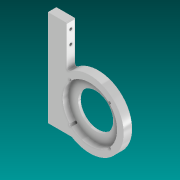
# Autodesk Inventor part: motorFrame
Saved by Autodesk Inventor 2020.3 (Build 243373000, 373)
## iProperties
Created: 2020-05-19
Part Number: motorFrame
Material: Aluminum 6061
Document SubType Name: Modeling
Designer: Svend
Density: 2.7 g/cm^3
Appearance: Aluminum - Polished
Author: Svend
Autodesk Inventor part; units mm, degrees
ref_plane "YZ Plane" through (0, 0, 0) normal (1, 0, 0) x (0, 1, 0)
ref_plane "XZ Plane" through (0, 0, 0) normal (0, 1, 0) x (-1, 0, 0)
ref_plane "Work Plane1" through (0, 0, 0) normal (0, 0, 1) x (1, 0, 0)
sketch "Sketch1" plane through (0, 0, 0) normal (0, 0, 1) x (1, 0, 0)
  circle A0 centre (0, 0) radius 21 projected
  circle A1 centre (23.57, -23.57) radius 2 projected
  circle A2 centre (23.57, 23.57) radius 2 projected
  circle A3 centre (-23.57, -23.57) radius 2.5 projected
  circle A4 centre (-23.57, 23.57) radius 2 projected
  circle A5 centre (-23.57, -23.57) radius 2 projected
  circle A6 centre (0, 0) radius 19 projected
  circle A7 centre (-23.57, 23.57) radius 2.5 projected
  circle A8 centre (-23.57, -23.57) radius 2.5 projected
  arc A9 (-29.95, -24.95) -> (-24.95, -29.95) centre (-24.95, -24.95) ccw projected
  line L0 (24.95, -29.95) -> (-24.95, -29.95) projected
  arc A10 (24.95, -29.95) -> (29.95, -24.95) centre (24.95, -24.95) ccw projected
  line L1 (29.95, 24.95) -> (29.95, -24.95) projected
  arc A11 (29.95, 24.95) -> (24.95, 29.95) centre (24.95, 24.95) ccw projected
  line L2 (-24.95, 29.95) -> (24.95, 29.95) projected
  arc A12 (-24.95, 29.95) -> (-29.95, 24.95) centre (-24.95, 24.95) ccw projected
  line L3 (-29.95, -24.95) -> (-29.95, 24.95) projected
  circle A13 centre (23.57, -23.57) radius 2.5 projected
  circle A14 centre (23.57, 23.57) radius 2.5 projected
  line L4 (-49.95, -90) -> (-49.95, 90) projected
  line L5 (-59.95, -90) -> (-49.95, -90)
  line L6 (-59.95, 90) -> (-49.95, 90)
  line L7 (40.2846, 0) -> (-40.2846, 0)
  line L8 (-49.95, -90) -> (-49.95, 90) projected
  line L9 (-59.95, -90) -> (-49.95, -90)
  line L10 (-49.95, 35.5095) -> (-26.95, 35.5095) projected
  line L11 (-24.95, 29.95) -> (-49.95, 29.95)
  line L12 (-24.95, -29.95) -> (-49.95, -29.95)
  circle A15 centre (0, 0) radius 22
  line L13 (-32.95, 22) -> (-32.95, -22) projected
  line L14 (-30.95, -14.95) -> (-49.95, -14.95)
  line L15 (-30.95, 14.95) -> (-49.95, 14.95)
  line L16 (-30.95, -14.95) -> (-30.95, 14.95)
  line L17 (24.7214, -34.026) -> (0, -42.0585)
  line L18 (0, -42.0585) -> (-24.7214, -34.026)
  line L19 (-24.7214, -34.026) -> (-40, -12.9968)
  line L20 (-40, -12.9968) -> (-40, 12.9968)
  line L21 (-40, 12.9968) -> (-24.7214, 34.026)
  line L22 (-24.7214, 34.026) -> (0, 42.0585)
  line L23 (0, 42.0585) -> (24.7214, 34.026)
  line L24 (24.7214, 34.026) -> (40, 12.9968)
  line L25 (40, 12.9968) -> (40, -12.9968)
  line L26 (40, -12.9968) -> (24.7214, -34.026)
  line L27 (-24.7214, -34.026) -> (-49.95, -34.026)
  line L28 (-24.7214, 34.026) -> (-49.95, 34.026)
  arc A16 (-24.7214, -34.026) -> (-24.7214, 34.026) centre (0, 0) ccw projected
  line L29 (-24.7214, 34.026) -> (-27.8, 34.026) projected
  line L30 (-27.8, 34.026) -> (-27.8, 80.5095) projected
  line L31 (-27.8, 80.5095) -> (-49.95, 80.5095) projected
  line L32 (-49.95, 80.5095) -> (-49.95, 14.95) projected
  line L33 (-49.95, 14.95) -> (-35.95, 14.95) projected
  arc A17 (-30.95, 9.95) -> (-35.95, 14.95) centre (-35.95, 9.95) ccw projected
  line L34 (-30.95, 9.95) -> (-30.95, -9.95) projected
  arc A18 (-35.95, -14.95) -> (-30.95, -9.95) centre (-35.95, -9.95) ccw projected
  line L35 (-35.95, -14.95) -> (-49.95, -14.95) projected
  line L36 (-49.95, -14.95) -> (-49.95, -34.026) projected
  line L37 (-49.95, -34.026) -> (-24.7214, -34.026) projected
  circle A19 centre (15.9909, -0.539) radius 1.6 projected
  circle A20 centre (-11.6884, -10.9261) radius 2 projected
  circle A21 centre (11.6884, 10.9261) radius 2 projected
  circle A22 centre (10.9261, -11.6884) radius 2 projected
  circle A23 centre (-15.9909, 0.539) radius 1.6 projected
  circle A24 centre (-0.539, -15.9909) radius 1.6 projected
  circle A25 centre (0, 0) radius 12.5 projected
  circle A26 centre (0.539, 15.9909) radius 1.6 projected
  circle A27 centre (-10.9261, 11.6884) radius 2 projected
  point P0 (0, 0)
  point P1 (-23.2856, -45.1645)
  point P2 (-49.95, -75.9684)
  point P3 (-23.2856, 45.1645)
  point P4 (-49.95, -14.95)
  point P5 (-32.95, 13.95)
  point P6 (-32.95, 14.95)
  dimension "d9" = 1
  dimension "d10" = 15
  dimension "d11" = 15
  dimension "d12" = 1
  dimension "d13" = 40
  constraints: 42 end point, 7 horizontal, 5 parallel, 2 perpendicular, 1 centre point, 1 coincident, 1 midpoint, 1 point on line, 1 symmetric about line, 1 vertical, 30 other
  measures "d9" radial gap between concentric circles of A0 A15
  measures "d10" distance between parallel lines of L12 L14
  measures "d11" distance between parallel lines of L11 L15
  measures "d12" distance between parallel lines of L3 L16
  measures "d13" distance from line of L25 point (0, 0)
extrude "Extrusion1" add sketch "Sketch1" along normal blind 10 contours L7 A15 A0 | A0 L7 A15 | A15 L7 L3 A12 L2 A11 L1 | L7 L1 A10 L0 A9 L3 A15 | L7 L25 L26 L17 L18 L19 L12 L0 A10 L1 | L1 A11 L2 L11 L21 L22 L23 L24 L25 L7 | L7 L16 L15 L21 L11 A12 L3 | L3 A9 L12 L19 L14 L16 L7 | L25 A16 | L16 A18 L13 L7 | L7 L13 A17 L16 | L24 A16 | A16 L26 | L13 A18 L14 L19 L20 L7 | L7 L20 L21 L15 A17 L13 | L16 L14 L13 A18 | A17 L13 L15 L16 | L23 A16 | A16 L17 | L19 L27 L4 L12 | L12 L4 L14 L19 | L21 L15 L4 L11 | L11 L4 L28 L21 | L20 L19 L14 L4 L15 L21 | A17 L15 L13 | L13 L14 A18 | L22 A16 | A16 L18 | A1 | A2 | A3 | A4 | A5 | A7 | A13 | A14
sketch "Sketch2" plane through (-49.95, -34.026, 0) normal (-1, 0, 0) x (0, 0, 1)
  line L0 (0, 68.0521) -> (0, 0) projected
  line L1 (0, 0) -> (10, 0) projected
  line L2 (10, 68.0521) -> (10, 0) projected
  line L3 (0, 68.0521) -> (0, 0) projected
  line L4 (10, 68.0521) -> (10, 0) projected
  line L5 (0, 68.0521) -> (10, 68.0521) projected
  line L6 (0, 0) -> (10, 0) projected
  line L7 (0, 68.0521) -> (10, 68.0521) projected
  point P0 (0, 34.026)
  point P1 (5, 7.5)
  point P2 (5, 60.5521)
  point P3 (5, 68.0521)
  point P4 (5, 19.076)
  dimension "d24" = 7.5
  dimension "d25" = 7.5
  constraints: 2 vertical alignment, 1 midpoint
  measures "d24" distance from line of L1 point (5, 7.5)
  measures "d25" distance from line of L5 point (5, 60.552)
hole "Hole1" at (-49.95, 26.526, 5) at (-49.95, -26.526, 5) direction (1, 0, 0) diameter 3.242 depth 15 tip angle 118 thread size "M4x0.7" class "6H" standard "ISO Metric profile"
sketch "Sketch3" plane through (0, 0, 10) normal (0, 0, 1) x (1, 0, 0)
  arc A0 (-24.7214, -34.026) -> (-24.7214, 34.026) centre (0, 0) ccw projected
  line L0 (-24.7214, 34.026) -> (-27.8, 34.026) projected
  line L1 (-27.8, 34.026) -> (-27.8, 80.5095) projected
  line L2 (-27.8, 80.5095) -> (-49.95, 80.5095) projected
  line L3 (-49.95, 80.5095) -> (-49.95, 14.95) projected
  line L4 (-49.95, 14.95) -> (-35.95, 14.95) projected
  arc A1 (-30.95, 9.95) -> (-35.95, 14.95) centre (-35.95, 9.95) ccw projected
  line L5 (-30.95, 9.95) -> (-30.95, -9.95) projected
  arc A2 (-35.95, -14.95) -> (-30.95, -9.95) centre (-35.95, -9.95) ccw projected
  line L6 (-35.95, -14.95) -> (-49.95, -14.95) projected
  line L7 (-49.95, -14.95) -> (-49.95, -34.026) projected
  line L8 (-49.95, -34.026) -> (-24.7214, -34.026) projected
  circle A3 centre (15.9909, -0.539) radius 1.6 projected
  circle A4 centre (-11.6884, -10.9261) radius 2 projected
  circle A5 centre (11.6884, 10.9261) radius 2 projected
  circle A6 centre (10.9261, -11.6884) radius 2 projected
  circle A7 centre (-15.9909, 0.539) radius 1.6 projected
  circle A8 centre (-0.539, -15.9909) radius 1.6 projected
  circle A9 centre (0, 0) radius 12.5 projected
  circle A10 centre (0.539, 15.9909) radius 1.6 projected
  circle A11 centre (-10.9261, 11.6884) radius 2 projected
  circle A12 centre (0, 0) radius 19 projected
  circle A13 centre (-23.57, 23.57) radius 2.5 projected
  circle A14 centre (-23.57, -23.57) radius 2.5 projected
  arc A15 (-29.95, -24.95) -> (-24.95, -29.95) centre (-24.95, -24.95) ccw projected
  line L9 (24.95, -29.95) -> (-24.95, -29.95) projected
  arc A16 (24.95, -29.95) -> (29.95, -24.95) centre (24.95, -24.95) ccw projected
  line L10 (29.95, 24.95) -> (29.95, -24.95) projected
  arc A17 (29.95, 24.95) -> (24.95, 29.95) centre (24.95, 24.95) ccw projected
  line L11 (-24.95, 29.95) -> (24.95, 29.95) projected
  arc A18 (-24.95, 29.95) -> (-29.95, 24.95) centre (-24.95, 24.95) ccw projected
  line L12 (-29.95, -24.95) -> (-29.95, 24.95) projected
  circle A19 centre (23.57, -23.57) radius 2.5 projected
  circle A20 centre (23.57, 23.57) radius 2.5 projected
  arc A21 (-37.4079, -14.95) -> (-37.4079, 14.95) centre (0, 0) ccw
  line L13 (-27.8, 34.026) -> (-27.8, 29.155)
  line L14 (-49.95, -34.026) -> (-21.5657, -34.026)
  line L15 (-49.95, -34.026) -> (-24.7214, -34.026) projected
  point P0 (0, 0)
  point P1 (-24.7214, -34.026)
  constraints: 4 end point, 4 point on circle, 2 collinear, 2 point on line, 1 centre point, 1 coincident, 1 tangent
extrude "Extrusion2" cut sketch "Sketch3" against normal blind 10 contours L14 A21 L13 L0 A0
sketch "Sketch4" plane through (0, 0, 10) normal (0, 0, 1) x (1, 0, 0)
  arc A0 (-24.7214, -34.026) -> (-24.7214, 34.026) centre (0, 0) ccw projected
  line L0 (-24.7214, 34.026) -> (-27.8, 34.026) projected
  line L1 (-27.8, 34.026) -> (-27.8, 80.5095) projected
  line L2 (-27.8, 80.5095) -> (-49.95, 80.5095) projected
  line L3 (-49.95, 80.5095) -> (-49.95, 14.95) projected
  line L4 (-49.95, 14.95) -> (-35.95, 14.95) projected
  arc A1 (-30.95, 9.95) -> (-35.95, 14.95) centre (-35.95, 9.95) ccw projected
  line L5 (-30.95, 9.95) -> (-30.95, -9.95) projected
  arc A2 (-35.95, -14.95) -> (-30.95, -9.95) centre (-35.95, -9.95) ccw projected
  line L6 (-35.95, -14.95) -> (-49.95, -14.95) projected
  line L7 (-49.95, -14.95) -> (-49.95, -34.026) projected
  line L8 (-49.95, -34.026) -> (-24.7214, -34.026) projected
  circle A3 centre (15.9909, -0.539) radius 1.6 projected
  circle A4 centre (-11.6884, -10.9261) radius 2 projected
  circle A5 centre (11.6884, 10.9261) radius 2 projected
  circle A6 centre (10.9261, -11.6884) radius 2 projected
  circle A7 centre (-15.9909, 0.539) radius 1.6 projected
  circle A8 centre (-0.539, -15.9909) radius 1.6 projected
  circle A9 centre (0, 0) radius 12.5 projected
  circle A10 centre (0.539, 15.9909) radius 1.6 projected
  circle A11 centre (-10.9261, 11.6884) radius 2 projected
  line L9 (-49.95, -90) -> (-49.95, 90) projected
  line L10 (-59.95, 90) -> (-49.95, 90)
  line L11 (-49.95, -90) -> (-49.95, 90) projected
  line L12 (-27.8, 29.155) -> (-27.8, 34.026) projected
  line L13 (-27.8, 34.026) -> (-49.95, 34.026) projected
  line L14 (-49.95, 34.026) -> (-49.95, -34.026) projected
  line L15 (-49.95, -34.026) -> (-21.5657, -34.026) projected
  arc A12 (-21.5657, -34.026) -> (-27.8, 29.155) centre (0, 0) ccw projected
  circle A13 centre (0, 0) radius 21 projected
  point P0 (0, 0)
  constraints: 2 end point, 1 horizontal, 1 other
extrude "Extrusion3" add sketch "Sketch4" against normal blind 10 contours L13 L3 L2 L1
fillet "Fillet1" radius 2 2 edges at (-27.8, 29.155, 5) (-21.5657, -34.026, 5)
fillet "Fillet2" radius 1 1 edges at (-27.8, 80.5095, 5)
sketch "Sketch5" plane through (-27.8, 33.5015, 10) normal (1, 0, 0) x (0, 0, -1)
  arc A0 (8, 9.19) -> (10, 11.19) centre (8, 11.19) ccw projected
  line L0 (10, 49.19) -> (10, 11.19) projected
  arc A1 (10, 49.19) -> (8, 51.19) centre (8, 49.19) ccw projected
  line L1 (-60.5, 51.19) -> (8, 51.19) projected
  arc A2 (-60.5, 51.19) -> (-62.5, 49.19) centre (-60.5, 49.19) ccw projected
  line L2 (-62.5, 11.19) -> (-62.5, 49.19) projected
  arc A3 (-62.5, 11.19) -> (-60.5, 9.19) centre (-60.5, 11.19) ccw projected
  line L3 (8, 9.19) -> (-60.5, 9.19) projected
  circle A4 centre (-26.25, 30.19) radius 12.6 projected
  circle A5 centre (-26.25, 14.19) radius 2 projected
  arc A6 (-59.6, 14.79) -> (-55.4, 14.79) centre (-57.5, 14.79) ccw projected
  line L4 (-59.6, 45.59) -> (-59.6, 14.79) projected
  arc A7 (-55.4, 45.59) -> (-59.6, 45.59) centre (-57.5, 45.59) ccw projected
  line L5 (-55.4, 14.79) -> (-55.4, 45.59) projected
  circle A8 centre (-42.25, 30.19) radius 2 projected
  circle A9 centre (-37.5637, 18.8763) radius 1.5 projected
  circle A10 centre (-37.5637, 41.5037) radius 1.5 projected
  circle A11 centre (-14.9363, 18.8763) radius 1.5 projected
  arc A12 (7.1, 45.59) -> (2.9, 45.59) centre (5, 45.59) ccw projected
  line L6 (7.1, 14.79) -> (7.1, 45.59) projected
  arc A13 (2.9, 14.79) -> (7.1, 14.79) centre (5, 14.79) ccw projected
  line L7 (2.9, 45.59) -> (2.9, 14.79) projected
  circle A14 centre (-10.25, 30.19) radius 2 projected
  circle A15 centre (-14.9363, 41.5037) radius 1.5 projected
  circle A16 centre (-26.25, 46.19) radius 2 projected
  circle A17 centre (-57.5, 11.46) radius 1.621 projected
  circle A18 centre (-57.5, 26.86) radius 1.621 projected
  arc A19 (8, 9.19) -> (10, 11.19) centre (8, 11.19) ccw projected
  line L8 (10, 49.19) -> (10, 11.19) projected
  arc A20 (10, 49.19) -> (8, 51.19) centre (8, 49.19) ccw projected
  line L9 (-60.5, 51.19) -> (8, 51.19) projected
  arc A21 (-60.5, 51.19) -> (-62.5, 49.19) centre (-60.5, 49.19) ccw projected
  line L10 (-62.5, 11.19) -> (-62.5, 49.19) projected
  arc A22 (-62.5, 11.19) -> (-60.5, 9.19) centre (-60.5, 11.19) ccw projected
  line L11 (8, 9.19) -> (-60.5, 9.19) projected
  circle A23 centre (-26.25, 30.19) radius 12.6 projected
  circle A24 centre (-26.25, 14.19) radius 2 projected
  arc A25 (-59.6, 14.79) -> (-55.4, 14.79) centre (-57.5, 14.79) ccw projected
  line L12 (-59.6, 45.59) -> (-59.6, 14.79) projected
  arc A26 (-55.4, 45.59) -> (-59.6, 45.59) centre (-57.5, 45.59) ccw projected
  line L13 (-55.4, 14.79) -> (-55.4, 45.59) projected
  circle A27 centre (-42.25, 30.19) radius 2 projected
  circle A28 centre (-37.5637, 18.8763) radius 1.5 projected
  circle A29 centre (-37.5637, 41.5037) radius 1.5 projected
  circle A30 centre (-14.9363, 18.8763) radius 1.5 projected
  arc A31 (7.1, 45.59) -> (2.9, 45.59) centre (5, 45.59) ccw projected
  line L14 (7.1, 14.79) -> (7.1, 45.59) projected
  arc A32 (2.9, 14.79) -> (7.1, 14.79) centre (5, 14.79) ccw projected
  line L15 (2.9, 45.59) -> (2.9, 14.79) projected
  circle A33 centre (-10.25, 30.19) radius 2 projected
  circle A34 centre (-14.9363, 41.5037) radius 1.5 projected
  circle A35 centre (-26.25, 46.19) radius 2 projected
  arc A36 (8, 9.19) -> (10, 11.19) centre (8, 11.19) ccw projected
  line L16 (10, 49.19) -> (10, 11.19) projected
  arc A37 (10, 49.19) -> (8, 51.19) centre (8, 49.19) ccw projected
  line L17 (-60.5, 51.19) -> (8, 51.19) projected
  arc A38 (-60.5, 51.19) -> (-62.5, 49.19) centre (-60.5, 49.19) ccw projected
  line L18 (-62.5, 11.19) -> (-62.5, 49.19) projected
  arc A39 (-62.5, 11.19) -> (-60.5, 9.19) centre (-60.5, 11.19) ccw projected
  line L19 (8, 9.19) -> (-60.5, 9.19) projected
  circle A40 centre (-26.25, 30.19) radius 12.6 projected
  circle A41 centre (-26.25, 14.19) radius 2 projected
  arc A42 (-59.6, 14.79) -> (-55.4, 14.79) centre (-57.5, 14.79) ccw projected
  line L20 (-59.6, 45.59) -> (-59.6, 14.79) projected
  arc A43 (-55.4, 45.59) -> (-59.6, 45.59) centre (-57.5, 45.59) ccw projected
  line L21 (-55.4, 14.79) -> (-55.4, 45.59) projected
  circle A44 centre (-42.25, 30.19) radius 2 projected
  circle A45 centre (-37.5637, 18.8763) radius 1.5 projected
  circle A46 centre (-37.5637, 41.5037) radius 1.5 projected
  circle A47 centre (-14.9363, 18.8763) radius 1.5 projected
  arc A48 (7.1, 45.59) -> (2.9, 45.59) centre (5, 45.59) ccw projected
  line L22 (7.1, 14.79) -> (7.1, 45.59) projected
  arc A49 (2.9, 14.79) -> (7.1, 14.79) centre (5, 14.79) ccw projected
  line L23 (2.9, 45.59) -> (2.9, 14.79) projected
  circle A50 centre (-10.25, 30.19) radius 2 projected
  circle A51 centre (-14.9363, 41.5037) radius 1.5 projected
  circle A52 centre (-26.25, 46.19) radius 2 projected
  point P0 (10, -33.5015)
  point P1 (5, 22.29)
  point P2 (5, 38.09)
  dimension "d47" = 7.5
  dimension "d48" = 7.5
  constraints: 2 vertical alignment
  measures "d47" distance of point (5, 38.09) A48.centre
  measures "d48" distance of A49.centre point (5, 22.29)
hole "Hole2" at (-27.8, 55.7915, 5) at (-27.8, 71.5915, 5) direction (-1, 0, 0) diameter 3.242 depth 22.15 thread size "M4x0.7" class "6H" standard "ISO Metric profile"
sketch "Sketch7" plane through (0, 0, 10) normal (0, 0, 1) x (1, 0, 0)
  circle A0 centre (0, 0) radius 32.55
  dimension "d49" = 65.1
  constraints: 1 centre point, 1 coincident
  measures "d49" diameter of A0
extrude "Extrusion5" cut sketch "Sketch7" against normal blind 7
sketch "Sketch10" plane through (0, 0, 0) normal (0, 0, -1) x (-1, 0, 0)
  point P0 (0, 0)
  point P1 (-23.57, -23.57)
  point P2 (-23.57, 23.57)
  point P3 (23.57, 23.57)
  point P4 (23.57, -23.57)
hole "Hole3" at (23.57, -23.57, 0) at (23.57, 23.57, 0) at (-23.57, 23.57, 0) at (-23.57, -23.57, 0) direction (0, 0, 1) diameter 3.242 depth 12 tip angle 118 thread size "M4x0.7" class "6H" standard "ISO Metric profile"
equation "\"d11\" = d10"
equation "\"d25\" = d24"
equation "\"d48\" = d47"
body "Solid1"
